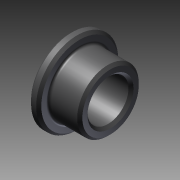
# Autodesk Inventor part: michaud_chailly_C2-151-8-128
Saved by Autodesk Inventor 2011 SP1 (Build 150282100, 282)
## iProperties
Created: 2015-04-11
Part Number: michaud_chailly_C2-151-8-128
Catalog Web Link: www.cadenas.de
Description: Modèle C2-151-Coussinet autolubrifiant à collerette - Alliage ferreux
Vendor: EMILEMAURIN
Document SubType Name: Modeling
Designer: PARTuser1
Manufacturer: EMILEMAURIN
Mass: 0.657213 g
Surface Area: 7.65867 cm^2
Volume: 0.657213 cm^3
Density: 1 g/cm^3
Category: PARTsolutions
Company: EMILEMAURIN
Title: Michaud Chailly C2-151-8-12-8
Author: Cadenas PARTsolutions
Comments: Coussinet autolubrifiant à collerette - Alliage ferreux
PSOL_IDENT_0: {$CADENAS_DATA\23d-libs\michaud_chailly_transmission\glissement\coussinets_autolubrifiants\collerett
PSOL_IDENT_1: e\c2_151.prj},211 {VTYP=3D},{NB=michaud_chailly_C2-151-8-128},{LINA=Michaud Chailly C2-151-8-12-8},{
PSOL_IDENT_2: NN=Modèle C2-151},{DATE=15.02.2013 07::03::32},{GEOMDATE=15.02.2013 07:01:42},{VERSION=},{LINEID=240
PSOL_IDENT_3: },{LINESUBID=-1},{WBVAR=L1}  {NB=michaud_chailly_C2-151-8-128},{LINA=Michaud Chailly C2-151-8-12-8},
PSOL_IDENT_4: {KT=DUMMY},{REF=C2-151-8-12},{MAT=Alliage ferreux},{D1=8},{D2=12},{D3=16},{L1=8},{L1X=8,12,16},{H1=2
PSOL_IDENT_5: .0},{INFOS=INFOTEXTE},{INFO1=c2_151.txt}
SUPPLIER: EMILEMAURIN
ARTICLENO: michaud_chailly_C2-151-8-128
BOMINFO: Michaud Chailly C2-151-8-12-8
CREATOR: CADENAS GmbH
Autodesk Inventor part; units mm, degrees
ref_plane "YZ Plane" through (0, 0, 0) normal (1, 0, 0) x (0, 1, 0)
ref_plane "XZ Plane" through (0, 0, 0) normal (0, 1, 0) x (-1, 0, 0)
ref_plane "XY Plane" through (0, 0, 0) normal (0, 0, 1) x (1, 0, 0)
sketch "Skizze_1" plane through (0, 0, 0) normal (0, 0, 1) x (1, 0, 0)
  line L0 (-2, 0) -> (6, 0)
  line L1 (-2, -7.5) -> (-1.5, -8)
  line L2 (-1.5, -8) -> (-0.5, -8)
  line L3 (-0.5, -8) -> (0, -7.5)
  line L4 (0, -7.5) -> (0, -6.5)
  arc A0 (0.5, -6) -> (0, -6.5) centre (0.5, -6.5) ccw
  line L5 (0.5, -6) -> (5.5, -6)
  line L6 (5.5, -6) -> (6, -5.5)
  line L7 (6, -5.5) -> (6, -4.5)
  line L8 (6, -4.5) -> (5.5, -4)
  line L9 (5.5, -4) -> (-1.5, -4)
  line L10 (-1.5, -4) -> (-2, -4.5)
  line L11 (-2, -4.5) -> (-2, -7.5)
  constraints: 24 end point, 2 point on circle, 1 centre point
revolve "Revolution1" add sketch "Skizze_1" angle 360 about axis through (-2, 0, 0) along (-1, 0, 0)
body "Solid1"
